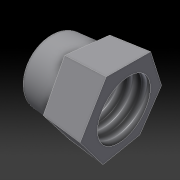
# Autodesk Inventor part: Hex Cap
Saved by Autodesk Inventor 2016 (Build 200138000, 138)
## iProperties
Created: 2012-08-08
Part Number: Hex Cap
Material: Generic
Document SubType Name: Modeling
Designer: John
Density: 1 g/cm^3
Appearance: Default
Author: John
Autodesk Inventor part; units mm, degrees
ref_plane "YZ Plane" through (0, 0, 0) normal (1, 0, 0) x (0, 1, 0)
ref_plane "XZ Plane" through (0, 0, 0) normal (0, 1, 0) x (-1, 0, 0)
ref_plane "XY Plane" through (0, 0, 0) normal (0, 0, 1) x (1, 0, 0)
sketch "Sketch1" plane through (0, 0, 0) normal (1, 0, 0) x (0, 1, 0)
  line L0 (3.556, -2.0531) -> (0, -4.1061)
  line L1 (0, -4.1061) -> (-3.556, -2.0531)
  line L2 (-3.556, -2.0531) -> (-3.556, 2.0531)
  line L3 (-3.556, 2.0531) -> (0, 4.1061)
  line L4 (0, 4.1061) -> (3.556, 2.0531)
  line L5 (3.556, 2.0531) -> (3.556, -2.0531)
  point P0 (0, 0)
  point P1 (0, 0)
  dimension "d0" = 7.112
  constraints: 12 end point, 1 coincident, 1 vertical, 13 other
  measures "d0" distance between parallel lines of L2 L5
extrude "Extrusion1" add sketch "Sketch1" along normal blind 3.429
sketch "Sketch2" plane through (0, 0, 0) normal (-1, 0, 0) x (0, 0, 1)
  circle A0 centre (0, 0) radius 3.4036
  dimension "d3" = 6.8072
  constraints: 1 centre point
  measures "d3" diameter of A0
extrude "Extrusion2" add sketch "Sketch2" along normal blind 3.175
sketch "Sketch3" plane through (-3.175, 0, 0) normal (-1, 0, 0) x (0, 0, 1)
  circle A0 centre (0, 0) radius 3.4036 projected
hole "Hole1" at (-3.175, 0, 0) direction (1, 0, 0) diameter 5.334 end through all
thread "Thread1" size "1/4-20 UNC" class "2B" standard "ANSI Unified Screw Threads" length 3.429 offset 3.175
body "Solid1"
